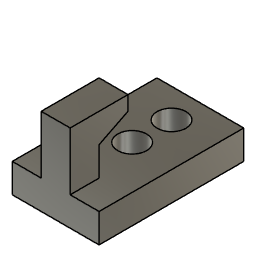
Halterung v3 (Autodesk Fusion 360 design; units mm, degrees)
Autodesk Fusion 360 part; units mm, degrees
sketch "Skizze1" plane through (0, 0, 0) normal (0, 0, 1) x (1, 0, 0)
  line L0 (0, 0) -> (15, 0)
  line L1 (15, 0) -> (15, -25)
  line L2 (15, -25) -> (0, -25)
  line L3 (0, -25) -> (0, 0)
  constraint horizontal L0
  constraint vertical L1
  constraint horizontal L2
  constraint vertical L3
  constraint coincident L0.start L3.end
extrude "Extrusion1" add sketch "Skizze1" along normal blind 5
sketch "Skizze2" plane through (0, 0, 5) normal (0, 0, 1) x (-1, 0, 0)
  line L0 (0, 25) -> (-15, 25)
  line L1 (-15, 25) -> (-15, 0)
  line L2 (-15, 0) -> (0, 0)
  line L3 (0, 0) -> (0, 25)
  line L4 (-5, 20) -> (-10, 20)
  line L5 (-10, 20) -> (-10, 25)
  line L6 (-10, 25) -> (-5, 25)
  line L7 (-5, 25) -> (-5, 20)
  dimension "d3" = 5
  constraint horizontal L4
  constraint vertical L5
  constraint horizontal L6
  constraint vertical L7
  measures "d3" distance of L4.start L4.end
extrude "Extrusion2" add sketch "Skizze2" along normal blind 10 contours L0 L4 L5 L6 L7
sketch "Skizze3" plane through (0, -20, 0) normal (0, 1, 0) x (-1, 0, 0)
  line L0 (-10, 5) -> (-5, 5)
  line L1 (-5, 5) -> (-5, 15)
  line L2 (-5, 15) -> (-10, 15)
  line L3 (-10, 15) -> (-10, 5)
  line L4 (-10, 15) -> (-5, 15)
  line L5 (-5, 15) -> (-5, 10)
  line L6 (-5, 10) -> (-10, 10)
  line L7 (-10, 10) -> (-10, 15)
  constraint horizontal L4
  constraint vertical L5
  constraint horizontal L6
  constraint vertical L7
  constraint midpoint L1 L5.end
  constraint coincident L2.end L3.start
extrude "Extrusion3" add sketch "Skizze3" along normal blind 5 contours L1 L2 L3 L4 L5 L6 L7
hole "Bohrung1" at (7.5542, -5.0286, 5) direction (0, 0, -1) diameter 5 depth 15 tip angle 118
hole "Bohrung2" at (7.5, -11.7857, 5) direction (0, 0, -1) diameter 5 depth 15 tip angle 118
sketch "Skizze4" plane through (5, 0, 0) normal (-1, 0, 0) x (0, -1, 0)
  line L0 (20, 5) -> (25, 5)
  line L1 (25, 5) -> (25, 15)
  line L2 (25, 15) -> (15, 15)
  line L3 (15, 15) -> (15, 10)
  line L4 (15, 10) -> (20, 10)
  line L5 (20, 10) -> (20, 5)
  line L6 (20, 10) -> (15, 12.5)
  line L7 (15, 10) -> (20, 10)
  constraint coincident L4.end L5.start
  constraint midpoint L3 L6.end
  constraint coincident L3.end L4.start
extrude "Extrusion4" cut sketch "Skizze4" against normal blind 5 contours L3 L4 L6 L7
